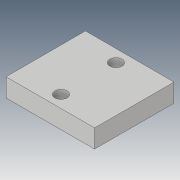
# Autodesk Inventor part: USB holder
Saved by Autodesk Inventor 2019 (Build 230136000, 136)
## iProperties
Created: 2020-09-21
Part Number: USB holder
Material: Generic
Document SubType Name: Modeling
Designer: giacomo
Density: 1 g/cm^3
Appearance: Default
Author: giacomo
Autodesk Inventor part; units mm, degrees
ref_plane "YZ Plane" through (0, 0, 0) normal (1, 0, 0) x (0, 1, 0)
ref_plane "XZ Plane" through (0, 0, 0) normal (0, 1, 0) x (-1, 0, 0)
ref_plane "XY Plane" through (0, 0, 0) normal (0, 0, 1) x (1, 0, 0)
sketch "Sketch1" plane through (0, 0, 0) normal (0, 1, 0) x (-1, 0, 0)
  line L0 (14.7043, 12.4547) -> (0.2043, 12.4547)
  line L1 (0.2043, 12.4547) -> (0.2043, -0.5453)
  line L2 (0.2043, -0.5453) -> (14.7043, -0.5453)
  line L3 (14.7043, -0.5453) -> (14.7043, 12.4547)
  line L4 (14.7043, 12.4547) -> (0.2043, -0.5453) construction
  line L5 (0.2043, 12.4547) -> (14.7043, -0.5453) construction
  point P0 (0, 0)
  point P1 (7.4543, 5.9547)
  dimension "d0" = 14.5
  dimension "d1" = 13
  constraints: 12 end point, 2 midpoint, 2 parallel, 1 horizontal, 1 perpendicular
  measures "d0" distance of L2.end L1.end
  measures "d1" distance of L1.end L0.end
extrude "Extrusion1" add sketch "Sketch1" along normal blind 3
sketch "Sketch2" plane through (0, 3, 0) normal (0, 1, 0) x (1, 0, 0)
  circle A0 centre (-7.7043, -10.4547) radius 1
  circle A1 centre (-7.7043, -1.4547) radius 1
  line L0 (-14.7043, -12.4547) -> (-0.2043, -12.4547) projected
  line L1 (-14.7043, 0.5453) -> (-14.7043, -12.4547) projected
  line L2 (-0.2043, 0.5453) -> (-14.7043, 0.5453) projected
  point P0 (0, 0)
  dimension "d4" = 2
  dimension "d5" = 2
  dimension "d6" = 2
  dimension "d7" = 7
  dimension "d8" = 7
  dimension "d9" = 2
  constraints: 2 centre point
  measures "d4" diameter of A0
  measures "d5" diameter of A1
  measures "d6" distance from line of L0 A0.centre
  measures "d7" distance from line of A0.centre L1
  measures "d8" distance from line of L1 A1.centre
  measures "d9" distance from line of L2 A1.centre
extrude "Extrusion2" cut sketch "Sketch2" against normal blind 3
body "Solid1"
